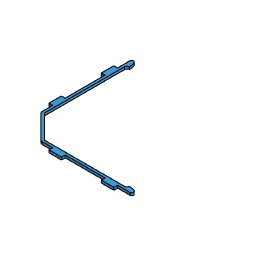
Tihend v4 (Autodesk Fusion 360 design; units mm, degrees)
Autodesk Fusion 360 part; units mm, degrees
sketch "Sketch1" plane through (0, 0, 0) normal (0, 0, 1) x (1, 0, 0)
  line L0 (-60.9778, -51.3602) -> (-51.369, -60.969)
  arc A0 (-51.369, -60.969) -> (-50.57, -61.3) centre (-50.57, -60.17) ccw
  line L1 (-50.8444, -61.3) -> (-15.6217, -61.3)
  arc A1 (-15.2933, -59.8758) -> (-17.7897, -59.3) centre (-17.7897, -65) ccw
  arc A2 (-18.7897, -60.3) -> (-17.7897, -59.3) centre (-18.7897, -59.3) ccw
  line L2 (-18.7897, -60.3) -> (-50.8444, -60.3)
  arc A3 (-50.6619, -60.2619) -> (-50.57, -60.3) centre (-50.57, -60.17) ccw
  line L3 (-50.6619, -60.2619) -> (-60.2707, -50.6531)
  arc A4 (-60.3, -50.5824) -> (-60.2707, -50.6531) centre (-60.2, -50.5824) ccw
  line L4 (-60.3, -50.8444) -> (-60.3, -18.8024)
  arc A5 (-59.3, -17.8024) -> (-60.3, -18.8024) centre (-59.3, -18.8024) ccw
  arc A6 (-59.3, -17.8024) -> (-59.8758, -15.306) centre (-65, -17.8024) ccw
  line L5 (-61.3, -15.6345) -> (-61.3, -50.8444)
  arc A7 (-61.3, -50.5824) -> (-60.9778, -51.3602) centre (-60.2, -50.5824) ccw
  arc A8 (-15.6217, -61.3) -> (-15.2933, -59.8758) centre (-15.6217, -60.55) ccw
  arc A9 (-59.8758, -15.306) -> (-61.3, -15.6345) centre (-60.55, -15.6345) ccw
  line L6 (-62.8, -15.6345) -> (-62.8, -50.8444)
  line L7 (-50.8444, -62.8) -> (-15.6217, -62.8)
  line L8 (-61.3, -46.5824) -> (-62.8, -46.5824)
  line L9 (-62.8, -41.5824) -> (-61.3, -41.5824)
  line L10 (-62.8, -20.5824) -> (-61.3, -20.5824)
  line L11 (-62.8, -25.5824) -> (-61.3, -25.5824)
  line L12 (-46.57, -61.3) -> (-46.57, -62.8)
  line L13 (-41.57, -61.3) -> (-41.57, -62.8)
  line L14 (-25.57, -61.3) -> (-25.57, -62.8)
  line L15 (-20.57, -61.3) -> (-20.57, -62.8)
  arc A10 (-51.6222, -60.9778) -> (-50.8444, -61.3) centre (-50.8444, -60.2) ccw
  line L16 (-60.9778, -51.6222) -> (-51.6222, -60.9778)
  arc A11 (-61.3, -50.8444) -> (-60.9778, -51.6222) centre (-60.2, -50.8444) ccw
  arc A12 (-60.3, -50.8444) -> (-60.2707, -50.9151) centre (-60.2, -50.8444) ccw
  line L17 (-50.9151, -60.2707) -> (-60.2707, -50.9151)
  arc A13 (-50.9151, -60.2707) -> (-50.8444, -60.3) centre (-50.8444, -60.2) ccw
  dimension "d1" = 60.3
  dimension "d2" = 60.3
  dimension "d3" = 1
  dimension "d4" = 1
  dimension "d5" = 1
  dimension "d6" = 5.7
  dimension "d7" = 0.75
  dimension "d8" = 3.7
  dimension "d9" = 1.13
  dimension "d10" = 1.1
  dimension "d11" = 45
  dimension "d12" = 50.57
  dimension "d13" = 31.7803
  dimension "d14" = 1
  dimension "d15" = 31.78
  dimension "d16" = 1
  dimension "d17" = 5.7
  dimension "d18" = 3.7
  dimension "d19" = 1
  dimension "d21" = 0.75
  dimension "d22" = 1.5
  dimension "d23" = 1.5
  dimension "d24" = 4
  dimension "d25" = 4
  dimension "d26" = 5
  dimension "d27" = 5
  dimension "d28" = 16
  dimension "d29" = 5
  dimension "d30" = 16
  dimension "d31" = 5
  constraint vertical L5
  constraint vertical L4
  constraint horizontal L2
  constraint horizontal L1
  constraint tangent L4 A5
  constraint tangent L5 A7
  constraint tangent L0 A7
  constraint tangent L0 A0
  constraint tangent A0 L1
  constraint tangent A2 L2
  constraint tangent L1 A8
  constraint tangent A1 A8
  constraint tangent L2 A3
  constraint tangent A3 L3
  constraint tangent A4 L4
  constraint tangent L3 A4
  constraint tangent A6 A9
  constraint tangent L5 A9
  constraint coincident L5 L8.start
  constraint coincident L6 L8.end
  constraint perpendicular L6 L8
  constraint coincident L6 L9.start
  constraint coincident L5 L9.end
  constraint perpendicular L5 L9
  constraint coincident L6 L10.start
  constraint coincident L5 L10.end
  constraint perpendicular L5 L10
  constraint coincident L6 L11.start
  constraint coincident L5 L11.end
  constraint perpendicular L5 L11
  constraint coincident L1 L12.start
  constraint coincident L7 L12.end
  constraint perpendicular L7 L12
  constraint coincident L1 L13.start
  constraint coincident L7 L13.end
  constraint perpendicular L7 L13
  constraint coincident L1 L14.start
  constraint coincident L7 L14.end
  constraint perpendicular L7 L14
  constraint coincident L1 L15.start
  constraint coincident L7 L15.end
  constraint perpendicular L7 L15
  constraint coincident A7.start L5
  constraint coincident A4.start L4
  constraint coincident A0.end L1
  constraint coincident A3.end L2
  measures "d1" distance of origin L4
  measures "d2" distance of origin L2
  measures "d3" distance of L1 L2
  measures "d4" distance of L4 L5
  measures "d5" radius of A2
  measures "d6" radius of A1
  measures "d7" radius of A8
  measures "d8" distance of A1.centre L1
  measures "d9" radius of A0
  measures "d10" radius of A7
  measures "d11" angle of L0 L5
  measures "d12" horizontal distance of origin A0.centre
  measures "d13" horizontal distance of A2.centre A0.centre
  measures "d14" horizontal distance of A1.centre A2.centre
  measures "d15" vertical distance of A5.centre A4.centre
  measures "d16" radius of A5
  measures "d17" radius of A6
  measures "d18" distance of A6.centre L5
  measures "d19" vertical distance of A5.centre A6.centre
  measures "d21" radius of A9
  measures "d24" distance of A4.centre L8
  measures "d25" distance of A0.centre L12
  measures "d26" distance of L8 L9
  measures "d27" distance of L12 L13
  measures "d28" distance of L9 L11
  measures "d29" distance of L10 L11
  measures "d30" distance of L13 L14
  measures "d31" distance of L14 L15
extrude "Extrude1" add sketch "Sketch1" along normal blind 1 contours L0 A0 L1 A1 A2 L2 L4 A5 A6 L5 A7 A8 A9 A12 L17 A13 | L0 A0 L1 L5 A7 A10 L16 A11 | L5 L6 L8 L9 | L1 L7 L12 L13 | L5 L6 L10 L11 | L1 L7 L14 L15
